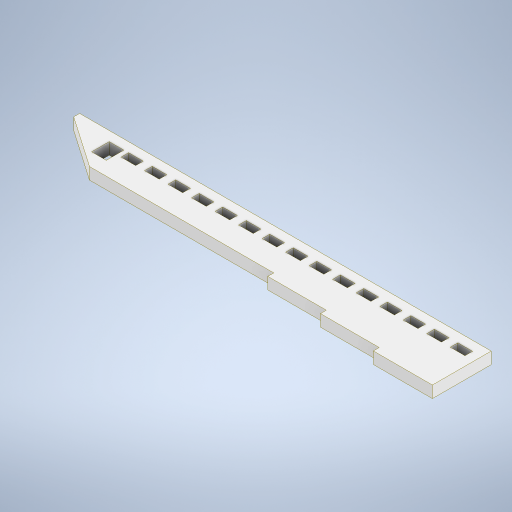
# Autodesk Inventor part: 援助旁邊4跟
Saved by Autodesk Inventor 2024.2 (Build 282272000, 272)
## iProperties
Created: 2024-06-02
Part Number: 援助旁邊4跟
Material: 一般
Document SubType Name: Modeling
Designer: sohil
Density: 1 g/cm^3
Appearance: 銀色
Author: sohil
Autodesk Inventor part; units mm, degrees
ref_plane "YZ Plane" through (0, 0, 0) normal (1, 0, 0) x (0, 1, 0)
ref_plane "XZ Plane" through (0, 0, 0) normal (0, 1, 0) x (-1, 0, 0)
ref_plane "XY Plane" through (0, 0, 0) normal (0, 0, 1) x (1, 0, 0)
sketch "草圖1" plane through (0, 0, 0) normal (0, 1, 0) x (-1, 0, 0)
  line L0 (21.4547, 24.4389) -> (-48.5453, 24.4389)
  line L1 (0.9998, 25.0567) -> (0.9998, 26.3567)
  line L2 (3.4998, 26.3567) -> (3.4998, 25.0567)
  line L3 (0.9998, 26.3567) -> (3.4998, 26.3567)
  line L4 (3.4998, 25.0567) -> (0.9998, 25.0567)
  line L5 (4.9998, 25.0567) -> (4.9998, 26.3567)
  line L6 (-18.5453, 30.4195) -> (12.788, 30.4195)
  line L7 (7.4998, 26.3567) -> (7.4998, 25.0567)
  line L8 (7.4998, 25.0567) -> (4.9998, 25.0567)
  line L9 (4.9998, 26.3567) -> (7.4998, 26.3567)
  line L10 (8.9998, 25.0567) -> (8.9998, 26.3567)
  line L11 (8.9998, 26.3567) -> (11.4998, 26.3567)
  line L12 (-48.5453, 23.4389) -> (-48.5453, 33.4389)
  line L13 (-38.5108, 33.4389) -> (-38.5108, 32.4389)
  line L14 (-38.5108, 32.4389) -> (-28.5108, 32.4389)
  line L15 (-28.5108, 32.4389) -> (-28.5108, 31.4389)
  line L16 (-18.5453, 31.4389) -> (-18.5453, 30.4195)
  line L17 (-28.5108, 31.4389) -> (-18.5453, 31.4389)
  line L18 (11.4998, 25.0567) -> (8.9998, 25.0567)
  line L19 (-44.5002, 26.3567) -> (-44.5002, 25.0567)
  line L20 (-44.5002, 25.0567) -> (-47.0002, 25.0567)
  line L21 (11.4998, 26.3567) -> (11.4998, 25.0567)
  line L22 (-40.5002, 26.3567) -> (-40.5002, 25.0567)
  line L23 (-40.5002, 25.0567) -> (-43.0002, 25.0567)
  line L24 (-47.0002, 25.0567) -> (-47.0002, 26.3567)
  line L25 (-47.0002, 26.3567) -> (-44.5002, 26.3567)
  line L26 (-43.0002, 26.3567) -> (-40.5002, 26.3567)
  line L27 (-36.5002, 26.3567) -> (-36.5002, 25.0567)
  line L28 (-39.0002, 26.3567) -> (-36.5002, 26.3567)
  line L29 (-39.0002, 25.0567) -> (-39.0002, 26.3567)
  line L30 (-36.5002, 25.0567) -> (-39.0002, 25.0567)
  line L31 (-43.0002, 25.0567) -> (-43.0002, 26.3567)
  line L32 (-32.5002, 26.3567) -> (-32.5002, 25.0567)
  line L33 (-32.5002, 25.0567) -> (-35.0002, 25.0567)
  line L34 (-35.0002, 26.3567) -> (-32.5002, 26.3567)
  line L35 (-35.0002, 25.0567) -> (-35.0002, 26.3567)
  line L36 (-28.5002, 26.3567) -> (-28.5002, 25.0567)
  line L37 (-28.5002, 25.0567) -> (-31.0002, 25.0567)
  line L38 (-31.0002, 26.3567) -> (-28.5002, 26.3567)
  line L39 (-31.0002, 25.0567) -> (-31.0002, 26.3567)
  line L40 (-24.5002, 26.3567) -> (-24.5002, 25.0567)
  line L41 (-24.5002, 25.0567) -> (-27.0002, 25.0567)
  line L42 (-27.0002, 25.0567) -> (-27.0002, 26.3567)
  line L43 (-27.0002, 26.3567) -> (-24.5002, 26.3567)
  line L44 (-20.5002, 26.3567) -> (-20.5002, 25.0567)
  line L45 (-20.5002, 25.0567) -> (-23.0002, 25.0567)
  line L46 (-23.0002, 26.3567) -> (-20.5002, 26.3567)
  line L47 (-23.0002, 25.0567) -> (-23.0002, 26.3567)
  line L48 (-16.5002, 26.3567) -> (-16.5002, 25.0567)
  line L49 (-19.0002, 26.3567) -> (-16.5002, 26.3567)
  line L50 (-19.0002, 25.0567) -> (-19.0002, 26.3567)
  line L51 (-16.5002, 25.0567) -> (-19.0002, 25.0567)
  line L52 (-12.5002, 26.3567) -> (-12.5002, 25.0567)
  line L53 (-15.0002, 26.3567) -> (-12.5002, 26.3567)
  line L54 (-15.0002, 25.0567) -> (-15.0002, 26.3567)
  line L55 (-12.5002, 25.0567) -> (-15.0002, 25.0567)
  line L56 (-8.5002, 26.3567) -> (-8.5002, 25.0567)
  line L57 (-8.5002, 25.0567) -> (-11.0002, 25.0567)
  line L58 (-11.0002, 25.0567) -> (-11.0002, 26.3567)
  line L59 (-11.0002, 26.3567) -> (-8.5002, 26.3567)
  line L60 (-4.5002, 25.0567) -> (-7.0002, 25.0567)
  line L61 (-7.0002, 26.3567) -> (-4.5002, 26.3567)
  line L62 (-7.0002, 25.0567) -> (-7.0002, 26.3567)
  line L63 (-4.5002, 26.3567) -> (-4.5002, 25.0567)
  line L64 (-3.0002, 25.0567) -> (-3.0002, 26.3567)
  line L65 (-0.5002, 25.0567) -> (-3.0002, 25.0567)
  line L66 (-3.0002, 26.3567) -> (-0.5002, 26.3567)
  line L67 (-0.5002, 26.3567) -> (-0.5002, 25.0567)
  line L68 (-48.5453, 33.4389) -> (-38.5108, 33.4389)
  line L69 (21.4547, 24.4389) -> (12.788, 30.4195)
  line L70 (12.2792, 28.0771) -> (12.2792, 25.0771)
  line L71 (14.7792, 28.0771) -> (12.2792, 28.0771)
  line L72 (12.2792, 25.0771) -> (14.7792, 25.0771)
  line L73 (14.7792, 25.0771) -> (14.7792, 28.0771)
  line L74 (-48.5453, 33.4389) -> (-48.5453, 23.4389)
  line L75 (-48.5453, 23.4389) -> (-48.5453, 24.4389)
  line L76 (-48.5453, 24.4389) -> (21.4547, 24.4389)
  line L77 (21.4547, 24.4389) -> (21.4547, 23.4389)
  line L78 (21.4547, 23.4389) -> (-48.5453, 23.4389)
  point P0 (34.4342, -20.4461)
  dimension "d19" = 2.5
  dimension "d20" = 3
  dimension "d26" = 70
  dimension "d27" = 10
  constraints: 158 end point, 4 parallel, 2 perpendicular, 1 collinear, 1 horizontal, 1 point on line, 1 vertical
  measures "d19" distance of L72.end L72.start
  measures "d20" distance of L72.start L70.start
  measures "d26" distance of L69.start L0.end
  measures "d27" distance of L12.end L12.start
extrude "擠出1" add sketch "草圖1" along normal blind 2
